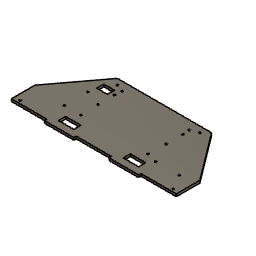
monitor_bottom_platef3d (Autodesk Fusion 360 design; units mm, degrees)
Autodesk Fusion 360 part; units mm, degrees
note: some values were not read from the file. Set by a fixed rule: the direction of a hole.
sketch "スケッチ1" plane through (0, 0, 0) normal (0, 1, 0) x (1, 0, 0)
  line L0 (-140, 0) -> (-80, 0)
  line L1 (-80, 0) -> (-80, -4)
  line L2 (-80, -4) -> (-30, -4)
  line L3 (-30, -4) -> (-30, 0)
  line L4 (-30, 0) -> (30, 0)
  line L5 (30, 0) -> (30, -4)
  line L6 (30, -4) -> (80, -4)
  line L7 (80, -4) -> (80, 0)
  line L8 (80, 0) -> (140, 0)
  line L9 (140, 0) -> (140, 40)
  line L10 (140, 40) -> (80, 120)
  line L11 (80, 120) -> (-80, 120)
  line L12 (-80, 120) -> (-140, 40)
  line L13 (-140, 40) -> (-140, 0)
  line L14 (-57, 105) -> (57, 105)
  line L15 (75, 30) -> (115, 30)
  line L16 (-85, 35) -> (-85, 75)
  line L17 (-70, 110) -> (70, 110)
  line L18 (-130, 5) -> (130, 5)
  line L19 (-57, 105) -> (-57, 35)
  line L20 (-57, 35) -> (57, 35)
  line L21 (57, 105) -> (57, 35)
  line L22 (-58, 65) -> (58, 65)
  line L23 (58, 65) -> (58, 93)
  line L24 (58, 93) -> (-58, 93)
  line L25 (-58, 93) -> (-58, 65)
  point P0 (0, 120)
  point P1 (0, 105)
  point P2 (0, 110)
  point P3 (0, 5)
  point P4 (0, 65)
  dimension "d1" = 280
  dimension "d2" = 60
  dimension "d3" = 50
  dimension "d4" = 4
  dimension "d5" = 80
  dimension "d6" = 40
  dimension "d7" = 160
  dimension "d22" = 114
  dimension "d23" = 15
  dimension "d27" = 40
  dimension "d28" = 30
  dimension "d29" = 25
  dimension "d30" = 40
  dimension "d31" = 35
  dimension "d32" = 55
  dimension "d36" = 140
  dimension "d37" = 10
  dimension "d38" = 5
  dimension "d39" = 260
  dimension "d40" = 70
  dimension "d41" = 116
  dimension "d42" = 28
  dimension "d43" = 65
  constraint horizontal L0
  constraint perpendicular L0 L1
  constraint perpendicular L1 L2
  constraint perpendicular L2 L3
  constraint perpendicular L3 L4
  constraint perpendicular L2 L5
  constraint perpendicular L3 L6
  constraint perpendicular L2 L7
  constraint perpendicular L7 L8
  constraint perpendicular L8 L9
  constraint perpendicular L7 L11
  constraint perpendicular L0 L13
  constraint midpoint L4 origin
  constraint midpoint L11 P0
  constraint vertical origin P0
  constraint equal L2 L6
  constraint equal L0 L8
  constraint collinear L2 L6
  constraint collinear L4 L8
  constraint collinear L0 L4
  constraint equal L9 L13
  constraint horizontal L14
  constraint midpoint L14 P1
  constraint vertical origin P1
  constraint horizontal L15
  constraint vertical L16
  constraint horizontal L17
  constraint midpoint L17 P2
  constraint vertical origin P2
  constraint horizontal L18
  constraint midpoint L18 P3
  constraint vertical origin P3
  constraint perpendicular L14 L19
  constraint perpendicular L19 L20
  constraint perpendicular L14 L21
  constraint coincident L20.end L21.end
  constraint horizontal L22
  constraint vertical L23
  constraint horizontal L24
  constraint vertical L25
  constraint midpoint L22 P4
  constraint vertical origin P4
  measures "d1" distance of L9 L13
  measures "d2" distance of L3.end L4.end
  measures "d3" distance of L1.end L2.end
  measures "d4" distance of L6.end L7.end
  measures "d5" vertical distance of L9.end L10.end
  measures "d6" distance of L8.end L9.end
  measures "d7" distance of L10.end L11.end
  measures "d22" distance of L14.start L14.end
  measures "d23" distance of L11 L14
  measures "d27" distance of L15.start L15.end
  measures "d28" distance of L8 L15
  measures "d29" distance of L9 L15.end
  measures "d30" distance of L16.start L16.end
  measures "d31" distance of L0 L16.start
  measures "d32" distance of L13 L16
  measures "d36" distance of L17.start L17.end
  measures "d37" distance of L11 L17
  measures "d38" distance of L0 L18
  measures "d39" distance of L18.start L18.end
  measures "d40" distance of L14.start L19.end
  measures "d41" distance of L23.end L24.end
  measures "d42" distance of L22.end L23.end
  measures "d43" distance of L4 L22
extrude "押し出し1" add sketch "スケッチ1" along normal blind 4 contours L0 L1 L2 L3 L4 L5 L6 L7 L8 L9 L10 L11 L12 L13 | L14 L19 L21 L24 | L19 L21 L22 L24 | L19 L22 L24 L25 | L21 L22 L23 L24 | L19 L20 L21 L22
hole "穴1" at (57, 0, -105) at (-57, 0, -105) at (-85, 0, -75) at (-85, 0, -35) at (75, 0, -30) at (115, 0, -30) at (-70, 0, -110) at (70, 0, -110) at (-130, 0, -5) at (130, 0, -5) at (-57, 0, -35) at (57, 0, -35) at (-58, 0, -93) at (-58, 0, -65) at (58, 0, -93) at (58, 0, -65) direction (0, 1, 0) diameter 3.2 end through all
sketch "スケッチ2" plane through (0, 4, 0) normal (0, 1, 0) x (-1, 0, 0)
  circle A0 centre (-58, -93) radius 1.6
  circle A1 centre (58, -93) radius 1.6
  circle A2 centre (57, -35) radius 1.6
  circle A3 centre (130, -5) radius 1.6
  circle A4 centre (70, -110) radius 1.6
  circle A5 centre (-75, -30) radius 1.6
  circle A6 centre (85, -75) radius 1.6
  circle A7 centre (-57, -105) radius 1.6
  circle A8 centre (57, -105) radius 1.6
  circle A9 centre (85, -35) radius 1.6
  circle A10 centre (-115, -30) radius 1.6
  circle A11 centre (-70, -110) radius 1.6
  circle A12 centre (-130, -5) radius 1.6
  circle A13 centre (-57, -35) radius 1.6
  circle A14 centre (58, -65) radius 1.6
  circle A15 centre (-58, -65) radius 1.6
  line L0 (140, -40) -> (140, 0)
  line L1 (140, 0) -> (80, 0)
  line L2 (80, 0) -> (80, 4)
  line L3 (80, 4) -> (30, 4)
  line L4 (30, 4) -> (30, 0)
  line L5 (30, 0) -> (-30, 0)
  line L6 (-30, 0) -> (-30, 4)
  line L7 (-30, 4) -> (-80, 4)
  line L8 (-80, 4) -> (-80, 0)
  line L9 (-80, 0) -> (-140, 0)
  line L10 (-140, 0) -> (-140, -40)
  line L11 (-140, -40) -> (-80, -120)
  line L12 (-80, -120) -> (80, -120)
  line L13 (80, -120) -> (140, -40)
  line L14 (68, -8) -> (42, -8)
  line L15 (42, -8) -> (42, -20)
  line L16 (42, -20) -> (68, -20)
  line L17 (68, -20) -> (68, -8)
  line L18 (-42, -8) -> (-68, -8)
  line L19 (-68, -8) -> (-68, -20)
  line L20 (-68, -20) -> (-42, -20)
  line L21 (-42, -20) -> (-42, -8)
  line L22 (83, -100) -> (65, -100)
  line L23 (65, -100) -> (65, -88)
  line L24 (65, -88) -> (83, -88)
  line L25 (83, -88) -> (83, -100)
  line L26 (55, 4) -> (55, -8)
  line L27 (-55, 4) -> (-55, -8)
  dimension "d44" = 18
  dimension "d45" = 12
  dimension "d46" = 12
  dimension "d47" = 88
  dimension "d48" = 65
  dimension "d50" = 26
  constraint horizontal L14
  constraint vertical L15
  constraint horizontal L16
  constraint vertical L17
  constraint horizontal L18
  constraint vertical L19
  constraint horizontal L20
  constraint vertical L21
  constraint horizontal L22
  constraint vertical L23
  constraint horizontal L24
  constraint vertical L25
  constraint equal L16 L20
  constraint equal L17 L21
  constraint equal L17 L25
  constraint midpoint L3 L26.start
  constraint perpendicular L3 L26
  constraint midpoint L7 L27.start
  constraint perpendicular L7 L27
  constraint midpoint L14 L26.end
  constraint midpoint L18 L27.end
  constraint equal L26 L27
  measures "d44" distance of L22.start L22.end
  measures "d45" distance of L22.start L24.end
  measures "d46" distance of L26.start L26.end
  measures "d47" distance of L5 L24
  measures "d48" distance of origin L23
  measures "d50" distance of L15.end L16.end
extrude "押し出し2" cut sketch "スケッチ2" against normal through all contours L14 L15 L16 L17 | L18 L19 L20 L21 | L22 L23 L24 L25
